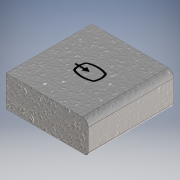
# Autodesk Inventor part: PRZYCISK IO
Saved by Autodesk Inventor 2017 SP1 (Build 210196100, 196)
## iProperties
Created: 2021-03-07
Part Number: PRZYCISK IO
Material: Tworzywo sztuczne, nieprzezroczyste czarne
Document SubType Name: Modeling
Designer: Administrator
Density: 0.952 g/cm^3
Appearance: Teksturowany - szary
Author: Administrator
Autodesk Inventor part; units mm, degrees
ref_plane "YZ Plane" through (0, 0, 0) normal (1, 0, 0) x (0, 1, 0)
ref_plane "XZ Plane" through (0, 0, 0) normal (0, 1, 0) x (-1, 0, 0)
ref_plane "XY Plane" through (0, 0, 0) normal (0, 0, 1) x (1, 0, 0)
sketch "Szkic1" plane through (0, 0, 0) normal (0, 0, 1) x (1, 0, 0)
  line L0 (206.45, -143.65) -> (206.45, -129.275)
  line L1 (206.45, -129.275) -> (220.2, -129.275)
  line L2 (206.45, -143.65) -> (220.2, -143.65)
  line L3 (220.2, -129.275) -> (220.2, -143.65)
  constraints: 8 end point
extrude "Wyciągnięcie proste1" add sketch "Szkic1" against normal blind 5.2
fillet "Zaokrąglenie1" radius 0.5 1 edges at (220.2, -136.4625, -5.2)
sketch "Szkic6" plane through (0, 0, 0) normal (0, 0, 1) x (1, 0, 0)
  arc A0 (214.7263, -135.514) -> (211.9237, -135.514) centre (213.325, -139.2478) ccw
  arc A1 (211.9237, -137.411) -> (214.7263, -137.411) centre (213.325, -133.6772) ccw
  arc A2 (214.8708, -137.2693) -> (214.8708, -135.6557) centre (212.8406, -136.4625) ccw
  arc A3 (211.9237, -135.514) -> (211.7792, -135.6557) centre (212.0023, -135.7386) ccw
  arc A4 (211.7792, -137.2693) -> (211.9237, -137.411) centre (212.0023, -137.1864) ccw
  arc A5 (214.8708, -135.6557) -> (214.7263, -135.514) centre (214.6477, -135.7386) ccw
  arc A6 (214.7263, -137.411) -> (214.8708, -137.2693) centre (214.6477, -137.1864) ccw
  arc A7 (213.325, -134.9597) -> (211.7797, -135.2472) centre (213.3235, -139.2481) ccw
  arc A8 (211.7797, -135.2472) -> (211.4912, -135.5391) centre (211.9597, -135.7137) ccw
  arc A9 (211.7797, -137.6778) -> (213.325, -137.9653) centre (213.3235, -133.6769) ccw
  arc A10 (211.4912, -137.3859) -> (211.7797, -137.6778) centre (211.9597, -137.2113) ccw
  arc A11 (213.325, -137.9653) -> (214.8703, -137.6778) centre (213.3265, -133.6769) ccw
  arc A12 (214.8703, -137.6778) -> (215.1588, -137.3859) centre (214.6903, -137.2113) ccw
  arc A13 (214.8703, -135.2472) -> (213.325, -134.9597) centre (213.3265, -139.2481) ccw
  arc A14 (215.1588, -135.5391) -> (214.8703, -135.2472) centre (214.6903, -135.7137) ccw
  arc A15 (215.1588, -137.3859) -> (215.1588, -135.5391) centre (212.6802, -136.4625) ccw
  line L0 (206.45, -143.65) -> (206.45, -129.275) projected
  line L1 (206.45, -129.275) -> (220.2, -129.275) projected
  line L2 (210.8247, -136.3625) -> (210.8247, -136.5625)
  line L3 (212.3974, -135.9987) -> (213.2356, -136.4178)
  line L4 (212.3974, -136.9263) -> (213.2356, -136.5072)
  line L5 (212.325, -136.0434) -> (212.325, -136.2625)
  line L6 (212.325, -136.6625) -> (212.325, -136.8816)
  arc A16 (212.3974, -135.9987) -> (212.325, -136.0434) centre (212.375, -136.0434) ccw
  arc A17 (212.325, -136.8816) -> (212.3974, -136.9263) centre (212.375, -136.8816) ccw
  arc A18 (213.2356, -136.5072) -> (213.2356, -136.4178) centre (213.2132, -136.4625) ccw
  arc A19 (210.8747, -136.3125) -> (210.8247, -136.3625) centre (210.8747, -136.3625) ccw
  arc A20 (210.8247, -136.5625) -> (210.8747, -136.6125) centre (210.8747, -136.5625) ccw
  arc A21 (212.275, -136.3125) -> (212.325, -136.2625) centre (212.275, -136.2625) ccw
  arc A22 (212.325, -136.6625) -> (212.275, -136.6125) centre (212.275, -136.6625) ccw
  arc A23 (211.7792, -135.6557) -> (211.6299, -136.3125) centre (213.8094, -136.4625) ccw
  arc A24 (211.6299, -136.6125) -> (211.7792, -137.2693) centre (213.8094, -136.4625) ccw
  arc A25 (211.4912, -135.5391) -> (211.329, -136.3125) centre (213.9698, -136.4625) ccw
  arc A26 (211.329, -136.6125) -> (211.4912, -137.3859) centre (213.9698, -136.4625) ccw
  line L7 (210.8747, -136.3125) -> (211.329, -136.3125)
  line L8 (211.6299, -136.3125) -> (212.275, -136.3125)
  line L9 (210.8747, -136.6125) -> (211.329, -136.6125)
  line L10 (211.6299, -136.6125) -> (212.275, -136.6125)
  point P0 (206.45, -136.4625)
  point P1 (213.325, -129.275)
  point P2 (210.8247, -136.3125)
  point P3 (210.8247, -136.6125)
  point P4 (212.325, -135.9625)
  point P5 (212.325, -136.9625)
  dimension "d70" = 0.3
  dimension "d75" = 1
  dimension "d78" = 0.05
  constraints: 54 point on circle, 27 centre point, 19 tangent, 18 end point, 8 perpendicular, 6 equal radius, 6 point on line, 3 vertical, 2 midpoint, 1 vertical alignment
  measures "d70" distance of point (210.825, -136.312) point (210.825, -136.612)
  measures "d75" distance of point (212.325, -135.962) point (212.325, -136.962)
  measures "d78" radius of A16
fillet "Zaokrąglenie2" radius 1 1 edges at (220.2, -136.4625, 0)
extrude "Wyciągnięcie proste5" add sketch "Szkic6" along normal blind 0.001
